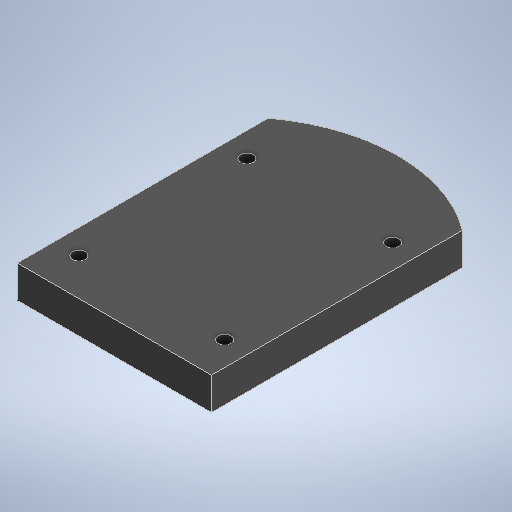
# Autodesk Inventor part: toe_sole_back
Saved by Autodesk Inventor 2026.1 (Build 301233020, 233B)
## iProperties
Created: 2024-02-12
Part Number: toe_sole_back
Material: 一般
Document SubType Name: Modeling
Designer: hibik
Density: 1 g/cm^3
Appearance: 既定
Author: hibik
Autodesk Inventor part; units mm, degrees
ref_plane "YZ Plane" through (0, 0, 0) normal (1, 0, 0) x (0, 1, 0)
ref_plane "XZ Plane" through (0, 0, 0) normal (0, 1, 0) x (-1, 0, 0)
ref_plane "XY Plane" through (0, 0, 0) normal (0, 0, 1) x (1, 0, 0)
sketch "スケッチ1" plane through (0, 0, 0) normal (0, 1, 0) x (-1, 0, 0)
  line L0 (26, 0) -> (0, 0)
  line L1 (0, 0) -> (0, -30)
  line L2 (0, -30) -> (26, -30)
  line L3 (26, -30) -> (26, 0)
  line L4 (26, 0) -> (27.9445, -37.1034)
  line L5 (0, 0) -> (-1.9445, -37.1034)
  arc A0 (-1.9445, -37.1034) -> (27.9445, -37.1034) centre (13, 0) ccw
  line L6 (0, 0) -> (26, -30)
  line L7 (0, -30) -> (26, 0)
  line L8 (4, -4.6154) -> (22, -4.6154)
  line L9 (22, -4.6154) -> (22, -25.3846)
  line L10 (22, -25.3846) -> (4, -25.3846)
  line L11 (4, -25.3846) -> (4, -4.6154)
  circle A1 centre (4, -4.6154) radius 0.8
  circle A2 centre (4, -25.3846) radius 0.8
  circle A3 centre (22, -4.6154) radius 0.8
  circle A4 centre (22, -25.3846) radius 0.8
  line L12 (38, 0) -> (-12, 0)
  line L13 (-12, 0) -> (-12, -40)
  line L14 (-12, -40) -> (38, -40)
  line L15 (38, -40) -> (38, 0)
  point P0 (13, -40)
  point P1 (13, -40)
  dimension "d0" = 26
  dimension "d3" = 30
  dimension "d4" = 3
  dimension "d5" = 3
  dimension "d6" = 40
  dimension "d17" = 4
  dimension "d18" = 1.6
  dimension "d19" = 1.6
  dimension "d20" = 1.6
  dimension "d21" = 1.6
  dimension "d28" = 50
  constraints: 32 end point, 6 coincident, 6 parallel, 5 centre point, 3 horizontal, 3 perpendicular, 3 point on line, 2 midpoint, 2 point on circle, 1 collinear, 1 tangent, 1 vertical alignment
  measures "d0" distance of L0.start L0.end
  measures "d3" distance of L2.end L0.start
  measures "d4" angle of L3 L4
  measures "d5" angle of L1 L5
  measures "d6" radius of A0
  measures "d17" distance between parallel lines of L1 L11
  measures "d18" diameter of A1
  measures "d19" diameter of A2
  measures "d20" diameter of A3
  measures "d21" diameter of A4
  measures "d28" distance of L13.end L14.end
extrude "押し出し1" add sketch "スケッチ1" along normal blind 1.5 contours L7 A3 L8 A1 L6 L0 | L4 A0 L5 L1 L2 L3 | L12 L15 L14 A0 L4 | L3 L6 A4 L9 A3 L7 | L6 A1 L11 A2 L7 L1 | L5 A0 L14 L13 L12 | L2 L7 A2 L10 A4 L6 | A3 L7 L6 A1 L8 | A1 L6 L7 A2 L11 | L10 A2 L7 L6 A4 | A3 L9 A4 L6 L7
sketch "スケッチ4" plane through (0, 0, 0) normal (0, -1, 0) x (1, 0, 0)
  line L0 (-38, 0) -> (12, 0) projected
  line L1 (-38, -40) -> (-38, 0) projected
  line L2 (12, -40) -> (-38, -40) projected
  line L3 (12, 0) -> (12, -40) projected
  circle A0 centre (-4, -25.3846) radius 0.8 projected
  circle A1 centre (-22, -25.3846) radius 0.8 projected
  circle A2 centre (-4, -4.6154) radius 0.8 projected
  circle A3 centre (-22, -4.6154) radius 0.8 projected
  circle A4 centre (-22, -4.6154) radius 2.5
  circle A5 centre (-4, -4.6154) radius 2.5
  circle A6 centre (-4, -25.3846) radius 2.5
  circle A7 centre (-22, -25.3846) radius 2.5
  line L4 (-36, -8) -> (-26, -8)
  line L5 (-26, -8) -> (-26, -38)
  line L6 (-26, -38) -> (-36, -38)
  line L7 (-36, -38) -> (-36, -8)
  line L8 (0, -8) -> (10, -8)
  line L9 (10, -8) -> (10, -38)
  line L10 (10, -38) -> (0, -38)
  line L11 (0, -38) -> (0, -8)
  point P0 (0, 0)
  dimension "d29" = 5
  dimension "d32" = 10
  dimension "d33" = 30
  dimension "d34" = 10
  dimension "d35" = 30
  dimension "d36" = 2
  dimension "d37" = 2
  dimension "d38" = 2
  constraints: 16 end point, 4 centre point, 4 coincident, 4 parallel, 3 equal radius, 2 horizontal, 2 perpendicular, 1 point on line
  measures "d29" diameter of A4
  measures "d32" distance of L5.end L6.end
  measures "d33" distance of L4.end L5.end
  measures "d34" distance of L9.end L10.end
  measures "d35" distance of L8.end L9.end
  measures "d36" distance between parallel lines of L3 L9
  measures "d37" distance between parallel lines of L1 L7
  measures "d38" distance between parallel lines of L2 L6
extrude "押し出し5" add sketch "スケッチ4" along normal blind 2.5 contours L0 L3 L2 L1
fillet "フィレット3" radius 1 8 edges at (-31, -2.5, -8) (-26, -2.5, -23) (-31, -2.5, -38) (-36, -2.5, -23) (0, -2.5, -23) (10, -2.5, -23) (5, -2.5, -8) (5, -2.5, -38)
sketch "スケッチ5" plane through (0, -2.5, 0) normal (0, -1, 0) x (1, 0, 0)
  line L0 (-1, -7) -> (-1, -39) projected
  line L1 (-25, -39) -> (-25, -7) projected
  line L2 (12, 0) -> (-38, 0) projected
  line L3 (-38, -40) -> (12, -40) projected
  line L4 (12, -40) -> (12, 0) projected
  line L5 (-38, 0) -> (-38, -40) projected
  line L6 (-1, 0) -> (-25, 0)
  line L7 (-25, 0) -> (-25, -40)
  line L8 (-25, -40) -> (-1, -40)
  line L9 (-1, -40) -> (-1, 0)
  arc A0 (-25, -31) -> (-1, -31) centre (-13, -15) ccw
  point P0 (0, 0)
  point P1 (-25, -7)
  point P2 (-1, -40)
  point P3 (-1, -31)
  point P4 (-25, -31)
  dimension "d42" = 20
  dimension "d43" = 15
  constraints: 8 end point, 6 point on line, 2 parallel, 2 point on circle, 1 centre point, 1 horizontal, 1 horizontal alignment, 1 perpendicular
  measures "d42" radius of A0
  measures "d43" distance from line of L2 A0.centre
extrude "押し出し6" cut sketch "スケッチ5" against normal through all contours L9 L2 L4 L3 L0 | L0 L9 L3 L7 L1 A0 | L1 L7 L3 L5 L2
sketch "スケッチ6" plane through (0, -2.5, 0) normal (0, -1, 0) x (1, 0, 0)
  line L0 (-3, -8.6154) -> (-5, -8.6154)
  line L1 (-5, -8.6154) -> (-5, -21.7082)
  line L2 (-5, -21.7082) -> (-3, -21.7082)
  line L3 (-3, -21.7082) -> (-3, -8.6154)
  line L4 (-8, -1) -> (-10, -1)
  line L5 (-10, -1) -> (-10, -25)
  line L6 (-10, -25) -> (-8, -25)
  line L7 (-8, -25) -> (-8, -1)
  circle A0 centre (-4, -4.6154) radius 0.8 projected
  circle A1 centre (-4, -25.3846) radius 0.8 projected
  line L8 (-1, 0) -> (-25, 0) projected
  arc A2 (-25.9808, -28.8744) -> (0.0379, -28.8208) centre (-13, -15) ccw
  arc A3 (-25, -31) -> (-1, -31) centre (-13, -15) ccw projected
  arc A4 (-25, -27.0416) -> (-1, -27.0416) centre (-13, -15) ccw
  line L9 (-1, -31) -> (-1, 0) projected
  line L10 (-25, -31) -> (-25, 0) projected
  line L11 (-2, -31.7033) -> (-2, -27.9615)
  line L12 (-24, -31.7033) -> (-24, -27.9615)
  circle A5 centre (-13, -15) radius 10.4403
  point P0 (0, 0)
  point P1 (-4, -8.6154)
  point P2 (-9, -1)
  point P3 (-24, -30.4919)
  point P4 (-2, -30.4919)
  point P5 (-8, -24.1652)
  point P6 (-3, -18)
  dimension "d44" = 2
  dimension "d45" = 4
  dimension "d47" = 1
  dimension "d48" = 24
  dimension "d49" = 3
  dimension "d52" = 1
  dimension "d53" = 2
  dimension "d54" = 1
  dimension "d55" = 1
  constraints: 20 end point, 10 point on circle, 6 parallel, 3 centre point, 2 concentric, 2 horizontal, 2 midpoint, 2 perpendicular, 2 point on line, 1 coincident, 1 vertical, 1 vertical alignment
  measures "d44" distance between parallel lines of L3 L1
  measures "d45" distance of A0.centre point (-4, -8.615)
  measures "d47" distance from line of L8 point (-9, -1)
  measures "d48" distance of L6.end L4.start
  measures "d49" distance between parallel lines of L1 L7
  measures "d52" radial gap between concentric circles of A3 A2
  measures "d53" radial gap between concentric circles of A2 A4
  measures "d54" distance between parallel lines of L9 L11
  measures "d55" distance between parallel lines of L10 L12
extrude "押し出し7" cut sketch "スケッチ6" against normal blind 0.8 contours L3 A5 L0 | A5 L3 L1 L0 | A5 L5 L4 L7 | L7 A5 L5 | L11 A2 L12 A4
ref_plane "作業平面1" through (-13, -2.5, 0) normal (1, 0, 0) x (0, 0, -1)
mirror "ミラー1" about plane through (-13, -2.5, 0) normal (1, 0, 0) of "押し出し7"
equation "\"d55\" = d54"
